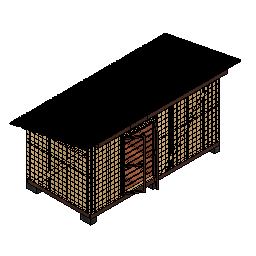
Сарай v19 (Autodesk Fusion 360 design; units mm, degrees)
Autodesk Fusion 360 part; units mm, degrees
note: some values were not read from the file. Chosen so that the rebuilt part matches the saved one: which bodies a step acts on; which face or edge a step refers to; where a step ends.
(part 1 of 2)
sketch "Sketch1" plane through (0, 0, 0) normal (0, 0, 1) x (1, 0, 0) in component "Обвязка"
  line L0 (0, 0) -> (5, 0)
  line L1 (5, 0) -> (5, 15)
  line L2 (5, 15) -> (0, 15)
  line L3 (0, 15) -> (0, 0)
  line L4 (0, 15) -> (-240, 15)
  line L5 (-240, 15) -> (-240, 0)
  line L6 (-240, 0) -> (0, 0)
  line L7 (0, 0) -> (0, 15)
  line L8 (-240, 15) -> (-245, 15)
  line L9 (-245, 15) -> (-245, 0)
  line L10 (-245, 0) -> (-240, 0)
  line L11 (-240, 0) -> (-240, 15)
  line L12 (-240, 15) -> (-235, 15)
  line L13 (-235, 15) -> (-235, 0)
  line L14 (-235, 0) -> (-240, 0)
  line L15 (-240, 0) -> (-240, 15)
  line L16 (0, 15) -> (-5, 15)
  line L17 (-5, 15) -> (-5, 0)
  line L18 (-5, 0) -> (0, 0)
  line L19 (0, 0) -> (0, 15)
  dimension "d1" = 5
  dimension "d2" = 15
  dimension "d3" = 240
  dimension "d4" = 15
  dimension "d5" = 5
  dimension "d6" = 15
  dimension "d7" = 5
  dimension "d8" = 15
  dimension "d9" = 5
  dimension "d10" = 15
  constraint horizontal L0
  constraint vertical L1
  constraint horizontal L2
  constraint vertical L3
  constraint coincident L0.start L3.end
  constraint horizontal L4
  constraint vertical L5
  constraint horizontal L6
  constraint vertical L7
  constraint horizontal L8
  constraint vertical L9
  constraint horizontal L10
  constraint vertical L11
  constraint horizontal L12
  constraint vertical L13
  constraint horizontal L14
  constraint vertical L15
  constraint horizontal L16
  constraint vertical L17
  constraint horizontal L18
  constraint vertical L19
  measures "d1" distance of L0.start L0.end
  measures "d2" distance of L0.start L2.end
  measures "d3" distance of L2.end L4.end
  measures "d4" distance of L2.end L0.start
  measures "d5" distance of L4.end L8.end
  measures "d6" distance of L4.end L5.end
  measures "d7" distance of L4.end L12.end
  measures "d8" distance of L4.end L5.end
  measures "d9" distance of L2.end L16.end
  measures "d10" distance of L2.end L0.start
extrude "Extrude1" add sketch "Sketch1" against normal blind 500 contours L0 L1 L2 L3 L7 L19 makes body 1 in component "Обвязка"
extrude "Extrude2" add sketch "Sketch1" against normal blind 500 separate body contours L5 L8 L9 L10 L11 L15 makes body 2 in component "Обвязка"
extrude "Extrude3" add sketch "Sketch1" against normal blind 5 separate body contours L3 L4 L6 L7 L16 L17 L18 L19 | L4 L6 L13 L17 | L4 L5 L6 L11 L12 L13 L14 L15 makes body 3 in component "Обвязка"
copy_body "CopyPasteBodies1" bodies 3 makes body 4 in component "Обвязка"
move_body "Move1" bodies 4 to x (1, 0, 0) y (0, 1, 0) z (0, 0, 1) at (0, 0, -495) in component "Обвязка"
extrude "Extrude4" add sketch "Sketch1" against normal blind 490 from surface at -5 separate body contours L3 L4 L6 L7 L16 L17 L18 L19 makes body 5 in component "Обвязка"
copy_body "CopyPasteBodies2" bodies 5 makes body 6 in component "Обвязка"
move_body "Move2" bodies 6 to x (1, 0, 0) y (0, 1, 0) z (0, 0, 1) at (-235, 0, 0) in component "Обвязка"
extrude "Extrude5" add sketch "Sketch1" against normal blind 5 from surface at -5 separate body contours L4 L6 L13 L17 makes body 7 in component "Обвязка"
copy_body "CopyPasteBodies3" bodies 7 makes body 8 in component "Обвязка"
move_body "Move3" bodies 8 to x (1, 0, 0) y (0, 1, 0) z (0, 0, 1) at (0, 0, -485) in component "Обвязка"
sketch "Sketch3" plane through (-235, 0, 0) normal (1, 0, 0) x (0, 0, -1) in component "Обвязка"
  line L0 (5, 15) -> (5, 0)
  line L1 (5, 0) -> (495, 0)
  line L2 (495, 0) -> (495, 15)
  line L3 (495, 15) -> (5, 15)
  point P0 (250, 15)
  constraint midpoint L3 P0
copy_body "CopyPasteBodies4" bodies 7 makes body 9 in component "Обвязка"
move_body "Move4" bodies 9 to x (1, 0, 0) y (0, 1, 0) z (0, 0, 1) at (0, 0, -240) in component "Обвязка"
copy_body "CopyPasteBodies5" bodies 9 makes body 10 in component "Обвязка"
move_body "Move5" bodies 10 to x (1, 0, 0) y (0, 1, 0) z (0, 0, 1) at (0, 0, -5) in component "Обвязка"
sketch "Sketch1 (2)" plane through (0, 0, 0) normal (0, 1, 0) x (1, 0, 0) in component "Фундамент"
  line L0 (-245, 0) -> (-205, 0)
  line L1 (-205, 0) -> (-205, 20)
  line L2 (-205, 20) -> (-245, 20)
  line L3 (-245, 20) -> (-245, 0)
  point P0 (-245, 0)
  dimension "d23" = 40
  dimension "d24" = 20
  constraint horizontal L0
  constraint vertical L1
  constraint horizontal L2
  constraint vertical L3
  constraint coincident P0 L0.start
  measures "d23" distance of P0 L0.end
  measures "d24" distance of P0 L2.end
extrude "Extrude1'" add sketch "Sketch1 (2)" against normal blind 20 separate body makes body 11 in component "Фундамент"
copy_body "CopyPasteBodies1'" bodies 11 makes body 12 in component "Фундамент"
move_body "Move1'" bodies 12 to x (1, 0, 0) y (0, 1, 0) z (0, 0, 1) at (210, 0, 0) in component "Фундамент"
copy_body "CopyPasteBodies2'" bodies 12 makes body 13 in component "Фундамент"
move_body "Move2'" bodies 13 to x (1, 0, 0) y (0, 1, 0) z (0, 0, 1) at (0, 0, -480) in component "Фундамент"
copy_body "CopyPasteBodies3'" bodies 11 makes body 14 in component "Фундамент"
move_body "Move3'" bodies 14 to x (1, 0, 0) y (0, 1, 0) z (0, 0, 1) at (0, 0, -480) in component "Фундамент"
copy_body "CopyPasteBodies4'" bodies 13 makes body 15 in component "Фундамент"
move_body "Move4'" bodies 15 to x (1, 0, 0) y (0, 1, 0) z (0, 0, 1) at (0, 0, 240) in component "Фундамент"
copy_body "CopyPasteBodies5'" bodies 15 makes body 16 in component "Фундамент"
move_body "Move5'" bodies 16 to x (1, 0, 0) y (0, 1, 0) z (0, 0, 1) at (-210, 0, 0) in component "Фундамент"
sketch "Sketch1 (3)" plane through (0, 0, 0) normal (0, 0, 1) x (1, 0, 0)
  line L0 (5, 15) -> (5, 295) construction
  line L1 (-245, 15) -> (-245, 295) construction
  line L2 (-302.9339, 205.9567) -> (-298.7516, 205.9567) construction
  line L3 (-298.7516, 205.9567) -> (44.8179, 272.7398) construction
  line L4 (-297.3309, 190.9521) -> (46.2386, 257.7352) construction
  point P0 (5, 15)
  point P1 (-245, 15)
  point P2 (5, 265)
  point P3 (5, 265)
  point P4 (5, 249.7192)
  point P5 (-245, 201.1242)
  point P6 (-245, 216.4049)
  dimension "d29" = 280
  dimension "d30" = 280
  dimension "d31" = 350
  dimension "d32" = 79
  dimension "d33" = 250
  dimension "d34" = 15
  constraint coincident P0 L0.start
  constraint vertical L0
  constraint coincident P1 L1.start
  constraint parallel L0 L1
  constraint perpendicular L1 L2
  constraint coincident L0 P3
  constraint coincident L3 P3
  constraint equal L3 L4
  constraint parallel L3 L4
  constraint coincident L4 P4
  constraint coincident L0 P4
  constraint coincident L4 P5
  constraint coincident L1 P5
  constraint coincident L1 P6
  constraint coincident L3 P6
  measures "d29" distance of P0 L0.end
  measures "d30" distance of P1 L1.end
  measures "d31" distance of L2.end L3.end
  measures "d32" angle of L0 L3
  measures "d33" distance of P0 P2
  measures "d34" distance of L3 L4
sketch "Sketch6" plane through (0, 0, 0) normal (0, 0, 1) x (1, 0, 0) in component "ЛицеваяСтена"
  line L0 (5, 15) -> (-5, 15)
  line L1 (-5, 15) -> (-5, 20)
  line L2 (-5, 20) -> (5, 20)
  line L3 (5, 20) -> (5, 15)
  line L4 (5, 15) -> (5, 264.9355) construction
  line L5 (5, 250.7192) -> (-5, 250.7192)
  line L6 (-5, 250.7192) -> (-5, 245.7192)
  line L7 (-5, 245.7192) -> (5, 245.7192)
  line L8 (5, 245.7192) -> (5, 250.7192)
  line L9 (5, 245.7192) -> (-5, 245.7192)
  line L10 (-5, 245.7192) -> (-5, 20)
  line L11 (-5, 20) -> (5, 20)
  line L12 (5, 20) -> (5, 245.7192)
  point P0 (5, 15)
  point P1 (5, 249.7192)
  point P2 (5, 250.7192)
  dimension "d42" = 10
  dimension "d43" = 5
  dimension "d44" = 1
  dimension "d45" = 10
  dimension "d46" = 5
  constraint horizontal L0
  constraint vertical L1
  constraint horizontal L2
  constraint vertical L3
  constraint coincident P0 L0.start
  constraint perpendicular L0 L4
  constraint coincident L4 P2
  constraint horizontal L5
  constraint vertical L6
  constraint horizontal L7
  constraint vertical L8
  constraint coincident P2 L5.start
  constraint horizontal L9
  constraint vertical L10
  constraint horizontal L11
  constraint vertical L12
  measures "d42" distance of P0 L0.end
  measures "d43" distance of P0 L2.end
  measures "d44" distance of P1 L5.start
  measures "d45" distance of P2 L5.end
  measures "d46" distance of P2 L7.end
extrude "Extrude2'" add sketch "Sketch6" against normal blind 500 separate body contours L0 L1 L2 L3 L11 makes body 17 in component "ЛицеваяСтена"
extrude "Extrude3'" add sketch "Sketch6" against normal blind 500 separate body contours L5 L6 L7 L8 L9 makes body 18 in component "ЛицеваяСтена"
extrude "Extrude4'" add sketch "Sketch6" against normal blind 5 separate body contours L2 L7 L9 L10 L11 L12 makes body 19 in component "ЛицеваяСтена"
pattern_linear "R-Pattern1" count 9 spacing 61.875 along (0, 0, -1) of bodies 19 makes body 20 at (-1.6667, 95.2397, -61.875) makes body 21 at (-1.6667, 95.2397, -123.75) makes body 22 at (-1.6667, 95.2397, -185.625) makes body 23 at (-1.6667, 95.2397, -247.5) makes body 24 at (-1.6667, 95.2397, -309.375) makes body 25 at (-1.6667, 95.2397, -371.25) makes body 26 at (-1.6667, 95.2397, -433.125) makes body 27 at (-1.6667, 95.2397, -495) in component "ЛицеваяСтена"
box "BoxPrimitive2" add length 250 width 125 height 1 placed x (0, 1, 0) y (0, 0, -1) z (-1, 0, 0) at (-5, 15, 0) separate body makes body 28 in component "ЛицеваяСтена"
sketch "Sketch9" plane through (5, 0, 0) normal (1, 0, 0) x (0, 0, -1) in component "ЛицеваяСтена"
  line L0 (0, 20) -> (0, 15)
  line L1 (0, 15) -> (500, 15)
  line L2 (500, 15) -> (500, 20)
  line L3 (500, 20) -> (0, 20)
  line L4 (120, 20) -> (120, 235) construction
  line L5 (255, 20) -> (255, 235) construction
  line L6 (120, 210) -> (255, 210) construction
  line L7 (120, 220) -> (255, 220) construction
  line L8 (185, 210) -> (185, 220) construction
  line L9 (0, 245.7192) -> (500, 245.7192)
  line L10 (492.3524, 260.7433) -> (289.7663, 14.3411) construction
  line L11 (467.0712, 253.613) -> (259.1771, 0.7549) construction
  line L12 (0, 250.7192) -> (500, 250.7192) construction
  line L13 (0, 20) -> (500, 20) construction
  line L14 (0, 15) -> (500, 15) construction
  line L15 (270.8891, 15) -> (290.308, 15)
  line L16 (290.308, 15) -> (484.1109, 250.7192)
  line L17 (484.1109, 250.7192) -> (464.692, 250.7192)
  line L18 (464.692, 250.7192) -> (270.8891, 15)
  point P0 (125, 20)
  point P1 (250, 20)
  point P2 (0, 20)
  point P3 (125, 20)
  point P4 (120, 20)
  point P5 (255, 20)
  point P6 (120, 210)
  point P7 (187.5, 210)
  point P8 (185, 210)
  point P9 (120, 220)
  point P10 (185, 220)
  point P11 (275, 20)
  point P12 (480, 245.7192)
  point P13 (495, 245.7192)
  point P14 (480, 245.7192)
  point P15 (275, 20)
  dimension "d67" = 125
  dimension "d68" = 125
  dimension "d69" = 5
  dimension "d70" = 5
  dimension "d71" = 215
  dimension "d72" = 215
  dimension "d73" = 190
  dimension "d79" = 2.5
  dimension "d80" = 10
  dimension "d96" = 20
  dimension "d97" = 15
  dimension "d98" = 15
  constraint coincident L3 P3
  constraint coincident L3 P1
  constraint coincident P2 L0.start
  constraint coincident P3 P0
  constraint coincident L3 P4
  constraint coincident L3 P5
  constraint coincident P4 L4.start
  constraint perpendicular L3 L4
  constraint coincident P5 L5.start
  constraint perpendicular L3 L5
  constraint coincident L4 P6
  constraint coincident P6 L6.start
  constraint coincident L5 L6.end
  constraint perpendicular L5 L6
  constraint midpoint L6 P7
  constraint coincident L6 P8
  constraint coincident L4 P9
  constraint coincident P9 L7.start
  constraint coincident L5 L7.end
  constraint perpendicular L5 L7
  constraint coincident P8 L8.start
  constraint coincident L7 P10
  constraint perpendicular L7 L8
  constraint coincident P10 L8.end
  constraint coincident L3 P15
  constraint coincident L9 P14
  constraint parallel L10 L11
  constraint coincident L10 P14
  constraint coincident L11 P15
  constraint coincident P14 P12
  constraint coincident P15 P11
  constraint coincident L11 L15.start
  constraint coincident L14 L15.start
  constraint coincident L10 L15.end
  constraint coincident L14 L15.end
  constraint coincident L10 L16.end
  constraint coincident L12 L16.end
  constraint coincident L11 L17.end
  constraint coincident L12 L17.end
  measures "d67" distance of P2 P3
  measures "d68" distance of P3 P1
  measures "d69" distance of P3 P4
  measures "d70" distance of P1 P5
  measures "d71" distance of P4 L4.end
  measures "d72" distance of P5 L5.end
  measures "d73" distance of P4 P6
  measures "d79" distance of P7 P8
  measures "d80" distance of P6 P9
  measures "d96" distance of P5 P15
  measures "d97" distance of P14 P13
  measures "d98" distance of L10 L11
move_body "Move2''" bodies 21 to x (1, 0, 0) y (0, 1, 0) z (0, 0, 1) at (0, 0, 3.75) in component "ЛицеваяСтена"
move_body "Move3''" bodies 23 to x (1, 0, 0) y (0, 1, 0) z (0, 0, 1) at (0, 0, -2.5) in component "ЛицеваяСтена"
move_body "Move4''" bodies 22 to x (1, 0, 0) y (0, 1, 0) z (0, 0, 1) at (0, 0, 70.625) in component "ЛицеваяСтена"
copy_body "CopyPasteBodies2''" bodies 22 makes body 29 in component "ЛицеваяСтена"
move_body "Move5''" bodies 29 to x (1, 0, 0) y (0, 1, 0) z (0, 0, 1) at (0, 0, -140) in component "ЛицеваяСтена"
box "BoxPrimitive4" add length 5 width 10 height 135 placed x (0, 1, 0) y (1, 0, 0) z (0, 0, -1) at (-5, 210.0714, -120) separate body makes body 30 in component "ЛицеваяСтена"
copy_body "CopyPasteBodies3''" bodies 30 makes body 31 in component "ЛицеваяСтена"
move_body "Move6" bodies 31 to x (1, 0, 0) y (0, 1, 0) z (0, 0, 1) at (0, 5, 0) in component "ЛицеваяСтена"
combine "Combine1" operation cut target body 21 tool bodies 30 31 keep tools makes body 32 at (-1.6667, 237.17, -120) in component "ЛицеваяСтена"
combine "Combine2" operation cut target body 23 tool bodies 30 31 keep tools makes body 33 at (-1.6667, 146.7143, -250) in component "ЛицеваяСтена"
copy_body "CopyPasteBodies4''" bodies 32 makes body 34 in component "ЛицеваяСтена"
move_body "Move7" bodies 34 to x (1, 0, 0) y (0, 1, 0) z (0, 0, 1) at (0, 0, -65) in component "ЛицеваяСтена"
sketch "Sketch1 (4)" plane through (0, 0, 0) normal (0, 0, 1) x (1, 0, 0) in component "ЗадняяСтена"
  line L0 (-245, 15) -> (-245, 230.3796) construction
  line L1 (-297.3309, 190.9521) -> (46.2386, 257.7352) construction
  line L2 (-245, 15) -> (-235, 15)
  line L3 (-235, 15) -> (-235, 20)
  line L4 (-235, 20) -> (-245, 20)
  line L5 (-245, 20) -> (-245, 15)
  line L6 (-235, 20) -> (-235, 230.5911) construction
  line L7 (-235, 204.068) -> (-245, 204.068)
  line L8 (-245, 204.068) -> (-245, 199.068)
  line L9 (-245, 199.068) -> (-235, 199.068)
  line L10 (-235, 199.068) -> (-235, 204.068)
  line L11 (-245, 199.068) -> (-235, 199.068)
  line L12 (-235, 199.068) -> (-235, 20)
  line L13 (-235, 20) -> (-245, 20)
  line L14 (-245, 20) -> (-245, 199.068)
  point P0 (-245, 15)
  point P1 (-245, 201.1242)
  point P2 (-235, 203.068)
  point P3 (-235, 204.068)
  dimension "d81" = 10
  dimension "d82" = 5
  dimension "d83" = 1
  dimension "d84" = 10
  dimension "d85" = 5
  constraint coincident P0 L0.start
  constraint vertical L0
  constraint horizontal L2
  constraint vertical L3
  constraint horizontal L4
  constraint vertical L5
  constraint perpendicular L4 L6
  constraint coincident L1 P2
  constraint coincident L6 P2
  constraint coincident L6 P3
  constraint horizontal L7
  constraint vertical L8
  constraint horizontal L9
  constraint vertical L10
  constraint coincident P3 L7.start
  constraint horizontal L11
  constraint vertical L12
  constraint horizontal L13
  constraint vertical L14
  measures "d81" distance of P0 L2.end
  measures "d82" distance of P0 L4.end
  measures "d83" distance of P2 P3
  measures "d84" distance of P3 L7.end
  measures "d85" distance of P3 L9.end
extrude "Extrude1''" add sketch "Sketch1 (4)" against normal blind 500 separate body contours L2 L3 L4 L5 L13 makes body 35 in component "ЗадняяСтена"
extrude "Extrude2''" add sketch "Sketch1 (4)" against normal blind 500 separate body contours L7 L8 L9 L10 L11 makes body 36 in component "ЗадняяСтена"
extrude "Extrude3''" add sketch "Sketch1 (4)" against normal blind 5 separate body contours L4 L9 L11 L12 L13 L14 makes body 37 in component "ЗадняяСтена"
sketch "Sketch2" plane through (-245, 0, 0) normal (-1, 0, 0) x (0, 0, 1) in component "ЗадняяСтена"
  line L0 (0, 15) -> (0, 20)
  line L1 (0, 20) -> (-500, 20)
  line L2 (-500, 20) -> (-500, 15)
  line L3 (-500, 15) -> (0, 15)
  line L4 (-185, 220.0714) -> (-185, 176.1812) construction
  line L5 (0, 199.068) -> (-500, 199.068) construction
  line L6 (0, 20) -> (-500, 20)
  line L7 (0, 199.068) -> (-500, 199.068)
  line L8 (0, 204.068) -> (-500, 204.068)
  line L9 (-466.0975, 206.5456) -> (-261.8081, 12.2071) construction
  line L10 (-487.598, 206.2959) -> (-282.9377, 11.6045) construction
  line L11 (-230.99, 2.9641) -> (-230.99, 3.2571) construction
  line L12 (-230.99, 3.2571) -> (-11.0284, 207.3942) construction
  line L13 (-22.6395, 217.0828) -> (-243.8333, 11.8022) construction
  line L14 (-485.256, 204.068) -> (-463.4929, 204.068)
  line L15 (-463.4929, 204.068) -> (-264.744, 15)
  line L16 (-264.744, 15) -> (-286.5071, 15)
  line L17 (-286.5071, 15) -> (-485.256, 204.068)
  line L18 (-240.3876, 15) -> (-218.3368, 15)
  line L19 (-218.3368, 15) -> (-14.6124, 204.068)
  line L20 (-14.6124, 204.068) -> (-36.6632, 204.068)
  line L21 (-36.6632, 204.068) -> (-240.3876, 15)
  point P0 (-125, 20)
  point P1 (-250, 20)
  point P2 (-185, 220.0714)
  point P3 (-185, 199.068)
  point P4 (-270, 20)
  point P5 (-235, 20)
  point P6 (-480, 199.068)
  point P7 (-20, 199.068)
  point P8 (-5, 199.068)
  point P9 (-480, 199.068)
  point P10 (-270, 20)
  point P11 (-20, 199.068)
  point P12 (-235, 20)
  point P13 (-247.5, 20)
  dimension "d103" = 20
  dimension "d104" = 15
  dimension "d105" = 20
  dimension "d106" = 15
  dimension "d107" = 15
  dimension "d108" = 15
  dimension "d173" = 252.5
  constraint coincident P2 L4.start
  constraint vertical L4
  constraint coincident L4 P3
  constraint coincident L5 P3
  constraint coincident L1 P10
  constraint coincident L1 P12
  constraint coincident L5 P9
  constraint coincident L5 P11
  constraint parallel L9 L10
  constraint coincident L10 P9
  constraint coincident L9 P10
  constraint coincident P9 P6
  constraint coincident P10 P4
  constraint perpendicular L3 L11
  constraint parallel L12 L13
  constraint coincident L12 P11
  constraint coincident L13 P12
  constraint coincident P11 P7
  constraint coincident P12 P5
  constraint coincident L10 L14.start
  constraint coincident L8 L14.start
  constraint coincident L9 L14.end
  constraint coincident L8 L14.end
  constraint coincident L9 L15.end
  constraint coincident L3 L15.end
  constraint coincident L3 L16.end
  constraint coincident L10 L16.end
  constraint coincident L3 L18.start
  constraint coincident L13 L18.start
  constraint coincident L12 L18.end
  constraint coincident L3 L18.end
  constraint coincident L8 L19.end
  constraint coincident L12 L19.end
  constraint coincident L13 L20.end
  constraint coincident L8 L20.end
  constraint coincident L1 P13
  measures "d103" distance of P1 P10
  measures "d104" distance of P1 P12
  measures "d105" distance of L5.end P9
  measures "d106" distance of P11 P8
  measures "d107" distance of L9 L10
  measures "d108" distance of L12 L13
  measures "d173" distance of L1.end P13
pattern_linear "R-Pattern1'" count 9 spacing 61.875 along (0, 0, -1) of bodies 37 makes body 38 at (-241.6667, 139.3787, -61.875) makes body 39 at (-241.6667, 139.3787, -123.75) makes body 40 at (-241.6667, 139.3787, -185.625) makes body 41 at (-241.6667, 139.3787, -247.5) makes body 42 at (-241.6667, 139.3787, -309.375) makes body 43 at (-241.6667, 139.3787, -371.25) makes body 44 at (-241.6667, 139.3787, -433.125) makes body 45 at (-241.6667, 139.3787, -495) in component "ЗадняяСтена"
move_body "Move1''" bodies 41 to x (1, 0, 0) y (0, 1, 0) z (0, 0, 1) at (0, 0, -2.5) in component "ЗадняяСтена"
move_body "Move2'''" bodies 39 to x (1, 0, 0) y (0, 1, 0) z (0, 0, 1) at (0, 0, 3.75) in component "ЗадняяСтена"
move_body "Move3'''" bodies 40 to x (1, 0, 0) y (0, 1, 0) z (0, 0, 1) at (0, 0, 0.625) in component "ЗадняяСтена"
extrude "Extrude5'" cut sketch "Sketch9" against normal blind 2.5 contours L3 L9 L16 L18 | L1 L3 L15 L16 L18 | L9 L16 L17 L18 bodies 17 18 24 25 26 in component "ЛицеваяСтена"
extrude "Extrude6" add sketch "Sketch9" against normal blind 2.5 separate body contours L3 L9 L16 L18 | L1 L3 L15 L16 L18 | L9 L16 L17 L18 makes body 46 in component "ЛицеваяСтена"
extrude "Extrude4''" cut sketch "Sketch2" against normal blind 2.5 contours L1 L3 L6 L18 L19 L21 | L1 L6 L7 L19 L21 | L7 L8 L19 L20 L21 | L1 L3 L6 L15 L16 L17 | L1 L6 L7 L15 L17 | L7 L8 L14 L15 L17 bodies 35 36 38 39 40 42 43 44 in component "ЗадняяСтена"
extrude "Extrude5''" add sketch "Sketch2" against normal blind 2.5 separate body contours L1 L3 L6 L15 L16 L17 | L1 L6 L7 L15 L17 | L7 L8 L14 L15 L17 makes body 47 in component "ЗадняяСтена"
extrude "Extrude6'" add sketch "Sketch2" against normal blind 2.5 separate body contours L1 L3 L6 L18 L19 L21 | L1 L6 L7 L19 L21 | L7 L8 L19 L20 L21 makes body 48 in component "ЗадняяСтена"
box "BoxPrimitive1" add length 5 width 10 height 230 placed x (0, 1, 0) y (0, 0, 1) z (1, 0, 0) at (-235, 15, -10) separate body makes body 49 in component "БоковаяСтена"
box "BoxPrimitive2'" add length 5 width 10 height 230 placed x (0, -1, 0) y (0, 0, -1) z (1, 0, 0) at (-235, 204.068, 0) separate body makes body 50 in component "БоковаяСтена"
sketch "Sketch3 (2)" plane through (0, 20, 0) normal (0, 1, 0) x (-1, 0, 0) in component "БоковаяСтена"
  line L0 (5, -10) -> (235, -10)
  line L1 (235, -10) -> (235, 0)
  line L2 (235, 0) -> (5, 0)
  line L3 (5, 0) -> (5, -10)
  line L4 (235, 0) -> (230, 0)
  line L5 (230, 0) -> (230, -10)
  line L6 (230, -10) -> (235, -10)
  line L7 (235, -10) -> (235, 0)
  dimension "d125" = 5
  dimension "d126" = 10
  constraint horizontal L4
  constraint vertical L5
  constraint horizontal L6
  constraint vertical L7
  constraint coincident L1.end L2.start
  measures "d125" distance of L1.end L4.end
  measures "d126" distance of L1.end L0.end
extrude "Extrude1'''" add sketch "Sketch3 (2)" along normal up to near side of body 50 separate body contours L0 L1 L2 L4 L5 L6 L7 makes body 51 in component "БоковаяСтена"
pattern_linear "R-Pattern1''" count 4 spacing 75 along (1, 0, 0) of bodies 51 makes body 52 at (-155, 79.6893, -3.3333) makes body 53 at (-80, 79.6893, -3.3333) makes body 54 at (-5, 79.6893, -3.3333) in component "БоковаяСтена"
sketch "Sketch4" plane through (0, 0, 0) normal (0, 0, 1) x (1, 0, 0) in component "БоковаяСтена"
  line L0 (-5, 20) -> (-235, 20)
  line L1 (-235, 20) -> (-235, 15)
  line L2 (-235, 15) -> (-5, 15)
  line L3 (-5, 15) -> (-5, 20)
  line L4 (-5, 204.068) -> (-235, 204.068)
  line L5 (-5, 199.068) -> (-235, 199.068)
  line L6 (-5, 20) -> (-235, 20)
  line L7 (-5, 15) -> (-235, 15)
  line L8 (-10.438, 214.4653) -> (-221.9216, -9.1487) construction
  line L9 (-27.6563, 218.0893) -> (-239.14, -5.5246) construction
  line L10 (-40.9171, 204.068) -> (-20.2712, 204.068)
  line L11 (-20.2712, 204.068) -> (-199.0829, 15)
  line L12 (-199.0829, 15) -> (-219.7288, 15)
  line L13 (-219.7288, 15) -> (-40.9171, 204.068)
  point P0 (-215, 20)
  point P1 (-25, 199.068)
  point P2 (-10, 199.068)
  point P3 (-230, 20)
  point P4 (-25, 199.068)
  point P5 (-215, 20)
  dimension "d133" = 15
  dimension "d134" = 15
  dimension "d135" = 15
  constraint coincident L0 P0
  constraint coincident L5 P4
  constraint parallel L8 L9
  constraint coincident L8 P4
  constraint coincident L9 P5
  constraint coincident P4 P1
  constraint coincident P0 P5
  constraint coincident L9 L10.start
  constraint coincident L4 L10.start
  constraint coincident L8 L10.end
  constraint coincident L4 L10.end
  constraint coincident L7 L11.end
  constraint coincident L8 L11.end
  constraint coincident L9 L12.end
  constraint coincident L7 L12.end
  measures "d133" distance of P4 P2
  measures "d134" distance of P0 P3
  measures "d135" distance of L8 L9
extrude "Extrude2'''" cut sketch "Sketch4" against normal blind 2.5 contours L0 L2 L6 L7 L11 L12 L13 | L0 L5 L6 L11 L13 | L4 L5 L10 L11 L13 bodies 49 50 52 53 in component "БоковаяСтена"
extrude "Extrude3'''" add sketch "Sketch4" against normal blind 2.5 separate body contours L0 L2 L6 L7 L11 L12 L13 | L0 L5 L6 L11 L13 | L4 L5 L10 L11 L13 makes body 55 in component "БоковаяСтена"
mirror "MirrorComponent1" about plane through (0, 0, 0) normal (0, 0, 1) of bodies 49 50 51 52 53 54 55 makes body 56 at (-68.118, 20, 4.1667) makes body 57 at (-170.3057, 204.068, 4.1667) makes body 58 at (-230, 79.6893, 3.3333) makes body 59 at (-155, 160.5258, 4.1667) makes body 60 at (-80, 60.3044, 4.1667) makes body 61 at (-5, 79.6893, 3.3333) makes body 62 at (-151.6667, 79.6893, 0) in component "БоковаяСтена(Mirror)"
sketch "Sketch1 (5)" plane through (-235, 0, 0) normal (1, 0, 0) x (0, 0, -1) in component "Лаги"
  line L0 (5, 15) -> (5, 0)
  line L1 (5, 0) -> (495, 0)
  line L2 (495, 0) -> (495, 15)
  line L3 (495, 15) -> (5, 15)
  line L4 (61.875, 20) -> (61.875, 0) construction
  line L5 (120, 20) -> (120, 0) construction
  line L6 (185, 20) -> (185, 0) construction
  line L7 (309.375, 20) -> (309.375, 0) construction
  line L8 (371.25, 20) -> (371.25, 0) construction
  line L9 (433.125, 20) -> (433.125, 0) construction
  line L10 (61.875, 15) -> (66.875, 15)
  line L11 (66.875, 15) -> (66.875, 5)
  line L12 (66.875, 5) -> (61.875, 5)
  line L13 (61.875, 5) -> (61.875, 15)
  point P0 (61.875, 20)
  point P1 (120, 20)
  point P2 (185, 20)
  point P3 (309.375, 20)
  point P4 (371.25, 20)
  point P5 (433.125, 20)
  point P6 (120, 15)
  point P7 (185, 15)
  point P8 (309.375, 15)
  point P9 (371.25, 15)
  point P10 (433.125, 15)
  point P11 (20, 15)
  point P12 (0, 15)
  point P13 (500, 15)
  point P14 (480, 15)
  dimension "d140" = 5
  dimension "d141" = 10
  dimension "d144" = 20
  dimension "d145" = 20
  constraint coincident P0 L4.start
  constraint coincident L1 L4.end
  constraint perpendicular L1 L4
  constraint coincident P1 L5.start
  constraint coincident L1 L5.end
  constraint perpendicular L1 L5
  constraint coincident P2 L6.start
  constraint coincident L1 L6.end
  constraint perpendicular L1 L6
  constraint coincident P3 L7.start
  constraint coincident L1 L7.end
  constraint perpendicular L1 L7
  constraint coincident P4 L8.start
  constraint coincident L1 L8.end
  constraint perpendicular L1 L8
  constraint coincident P5 L9.start
  constraint coincident L1 L9.end
  constraint perpendicular L1 L9
  constraint horizontal L10
  constraint vertical L11
  constraint horizontal L12
  constraint vertical L13
  constraint coincident L3 L10.start
  constraint coincident L4 L10.start
  constraint coincident L5 P6
  constraint coincident L3 P6
  constraint coincident L6 P7
  constraint coincident L3 P7
  constraint coincident L7 P8
  constraint coincident L3 P8
  constraint coincident L8 P9
  constraint coincident L3 P9
  constraint coincident L9 P10
  constraint coincident L3 P10
  constraint coincident L3 P11
  constraint coincident L3 P14
  measures "d140" distance of L10.start L10.end
  measures "d141" distance of L10.start L12.end
  measures "d144" distance of P11 P12
  measures "d145" distance of P13 P14
extrude "Extrude1''''" add sketch "Sketch1 (5)" along normal blind 230 separate body contours L3 L10 L11 L12 L13 makes body 63 in component "Лаги"
copy_body "CopyPasteBodies1''" bodies 63 makes body 64 in component "Лаги"
move_body "Move1'''" bodies 64 to x (1, 0, 0) y (0, 1, 0) z (0, 0, 1) at (0, 0, -58.125) in component "Лаги"
copy_body "CopyPasteBodies2'''" bodies 64 makes body 65 in component "Лаги"
move_body "Move2''''" bodies 65 to x (1, 0, 0) y (0, 1, 0) z (0, 0, 1) at (0, 0, -65) in component "Лаги"
copy_body "CopyPasteBodies3'''" bodies 65 makes body 66 in component "Лаги"
move_body "Move3''''" bodies 66 to x (1, 0, 0) y (0, 1, 0) z (0, 0, 1) at (0, 0, -124.375) in component "Лаги"
copy_body "CopyPasteBodies4'''" bodies 66 makes body 67 in component "Лаги"
move_body "Move4'''" bodies 67 to x (1, 0, 0) y (0, 1, 0) z (0, 0, 1) at (0, 0, -61.875) in component "Лаги"
copy_body "CopyPasteBodies5''" bodies 67 makes body 68 in component "Лаги"
move_body "Move5'''" bodies 68 to x (1, 0, 0) y (0, 1, 0) z (0, 0, 1) at (0, 0, -61.875) in component "Лаги"
copy_body "CopyPasteBodies6" bodies 63 makes body 69 in component "Лаги"
move_body "Move6'" bodies 69 to x (1, 0, 0) y (0, 1, 0) z (0, 0, 1) at (0, 0, 41.875) in component "Лаги"
copy_body "CopyPasteBodies7" bodies 68 makes body 70 in component "Лаги"
move_body "Move7'" bodies 70 to x (1, 0, 0) y (0, 1, 0) z (0, 0, 1) at (0, 0, -41.875) in component "Лаги"
sketch "Sketch1 (6)" plane through (0, 0, 0) normal (0, 0, 1) x (1, 0, 0) in component "Стропила"
  line L0 (-298.7516, 205.9567) -> (44.8179, 272.7398)
  line L1 (-297.3309, 190.9521) -> (46.2386, 257.7352)
  line L2 (-259.4542, 261.2143) -> (-259.4542, 7.593) construction
  line L3 (35, 295.2761) -> (35, -0.5469) construction
  line L4 (5, 15) -> (5, 295) construction
  line L5 (-259.4882, 213.5887) -> (-256.626, 198.8643)
  line L6 (-259.4882, 213.5887) -> (35, 270.8314)
  line L7 (35, 270.8314) -> (35, 255.5507)
  line L8 (35, 255.5507) -> (-256.626, 198.8643)
  line L9 (-245, 199.068) -> (-235, 199.068)
  line L10 (-235, 199.068) -> (-235, 204.068)
  line L11 (-235, 204.068) -> (-245, 204.068)
  line L12 (-245, 204.068) -> (-245, 199.068)
  line L13 (-245, 201.1242) -> (-245, 204.068)
  line L14 (-235, 204.068) -> (-234.9283, 203.0819)
  line L15 (-45.6459, 199.068) -> (-40.9171, 204.068)
  line L16 (-40.9171, 204.068) -> (-235, 204.068)
  line L17 (-235, 204.068) -> (-235, 199.068)
  line L18 (-235, 199.068) -> (-45.6459, 199.068)
  line L19 (-235, 204.068) -> (-229.8554, 204.068)
  point P0 (-259.4882, 213.5887)
  point P1 (35, 270.8314)
  dimension "d146" = 300
  dimension "d147" = 30
  constraint coincident L0 P0
  constraint coincident L0 P1
  constraint vertical L2
  constraint parallel L2 L3
  constraint coincident P1 L3
  constraint coincident P0 L5.start
  constraint coincident L1 L5.end
  constraint perpendicular L1 L5
  constraint coincident P1 L6.end
  constraint coincident L3 L7.end
  constraint coincident L1 L7.end
  constraint coincident L1 L13.start
  constraint coincident L12 L13.start
  constraint coincident L11.end L12.start
  constraint coincident L10.end L11.start
  constraint coincident L1 L14.end
  constraint coincident L8 L19.end
  constraint coincident L16 L19.end
  measures "d146" distance of P0 P1
  measures "d147" distance of L3 L4
extrude "Extrude1'''''" add sketch "Sketch1 (6)" against normal blind 5 separate body contours L0 L1 L5 L6 L7 L8 L11 L12 L13 L16 L19 | L1 L8 L14 L16 L19 makes body 71 in component "Стропила"
pattern_linear "R-Pattern1'''" count 9 spacing 61.875 along (0, 0, -1) of bodies 71 makes body 72 at (-151.4479, 229.496, -61.875) makes body 73 at (-151.4479, 229.496, -123.75) makes body 74 at (-151.4479, 229.496, -185.625) makes body 75 at (-151.4479, 229.496, -247.5) makes body 76 at (-151.4479, 229.496, -309.375) makes body 77 at (-151.4479, 229.496, -371.25) makes body 78 at (-151.4479, 229.496, -433.125) makes body 79 at (-151.4479, 229.496, -495) in component "Стропила"
sketch "Sketch2 (2)" plane through (-245, 0, 0) normal (-1, 0, 0) x (0, 0, 1) in component "Стропила"
  line L0 (-66.875, 176.0297) -> (-61.875, 180.6699)
  line L1 (-61.875, 180.6699) -> (-61.875, 199.068)
  line L2 (-61.875, 199.068) -> (-66.875, 199.068)
  line L3 (-66.875, 199.068) -> (-66.875, 176.0297)
  line L4 (-255, 199.068) -> (-255, 207.4684) construction
  line L5 (-120, 199.068) -> (-120, 207.4684) construction
  line L6 (-463.4929, 204.068) -> (-458.2369, 199.068) construction
  line L7 (-458.2369, 199.068) -> (-42.0508, 199.068) construction
  line L8 (-42.0508, 199.068) -> (-36.6632, 204.068) construction
  line L9 (-36.6632, 204.068) -> (-463.4929, 204.068) construction
  point P0 (-120, 199.068)
  point P1 (-255, 199.068)
  point P2 (-255, 204.068)
  point P3 (-120, 204.068)
  constraint coincident P1 L4.start
  constraint vertical L4
  constraint coincident P0 L5.start
  constraint parallel L4 L5
  constraint coincident L4 P2
  constraint coincident L9 P2
  constraint coincident L5 P3
  constraint coincident L9 P3
move_body "Move1''''" bodies 73 to x (1, 0, 0) y (0, 1, 0) z (0, 0, 1) at (0, 0, 3.75) in component "Стропила"
move_body "Move2'''''" bodies 75 to x (1, 0, 0) y (0, 1, 0) z (0, 0, 1) at (0, 0, -2.5) in component "Стропила"
combine "Combine1'" operation cut target body 71 tool bodies 50 keep tools in component "Стропила"
combine "Combine2'" operation cut target body 79 tool bodies 57 body 57 seen with x (1, 0, 0) y (0, 1, 0) z (0, 0, 1) at (0, 0, -500) keep tools in component "Стропила"
box "BoxPrimitive1'" add length 480 width 15 height 2.5 placed x (0, 0, -1) y (-1, 0, 0) z (0, 1, 0) at (-220, 15, -10) separate body makes body 80 in component "Пол"
pattern_linear "R-Pattern1''''" count 13 spacing 17.9167 along (1, 0, 0) of bodies 80 makes body 81 at (-212.0833, 15, -170) makes body 82 at (-194.1667, 15, -170) makes body 83 at (-176.25, 15, -170) makes body 84 at (-158.3333, 15, -170) makes body 85 at (-140.4167, 15, -170) makes body 86 at (-122.5, 15, -170) makes body 87 at (-104.5833, 15, -170) makes body 88 at (-86.6667, 15, -170) makes body 89 at (-68.75, 15, -170) makes body 90 at (-50.8333, 15, -170) makes body 91 at (-32.9167, 15, -170) makes body 92 at (-15, 15, -170) in component "Пол"
combine "Combine3" operation cut target body 71 tool bodies 18 keep tools in component "Стропила"
combine "Combine4" operation cut target body 72 tool bodies 18 keep tools in component "Стропила"
combine "Combine5" operation cut target body 73 tool bodies 18 keep tools in component "Стропила"
combine "Combine6" operation cut target body 74 tool bodies 18 keep tools in component "Стропила"
combine "Combine7" operation cut target body 75 tool bodies 18 keep tools in component "Стропила"
combine "Combine8" operation cut target body 76 tool bodies 18 keep tools in component "Стропила"
combine "Combine9" operation cut target body 77 tool bodies 18 keep tools in component "Стропила"
combine "Combine10" operation cut target body 78 tool bodies 18 keep tools in component "Стропила"
combine "Combine11" operation cut target body 79 tool bodies 18 keep tools in component "Стропила"
sketch "Sketch1 (7)" plane through (-49.4533, 254.4153, 0) normal (-0.190809, 0.981627, 0) x (0, 0, 1) in component "Обрешетка"
  line L0 (0, -213.966) -> (0, 86.034)
  line L1 (0, 86.034) -> (-5, 86.034)
  line L2 (-5, 86.034) -> (-5, -213.966)
  line L3 (-5, -213.966) -> (0, -213.966)
  line L4 (0, -213.966) -> (-500, -213.966) construction
  line L5 (-500, -213.966) -> (-500, -198.966) construction
  line L6 (-500, -198.966) -> (0, -198.966) construction
  line L7 (0, -198.966) -> (0, -213.966) construction
  line L8 (0, -198.966) -> (-500, -213.966) construction
  line L9 (-550, -198.966) -> (50, -198.966)
  line L10 (50, -198.966) -> (50, -213.966)
  line L11 (50, -213.966) -> (-550, -213.966)
  line L12 (-550, -213.966) -> (-550, -198.966)
  line L13 (-550, -198.966) -> (50, -213.966) construction
  line L14 (50, -198.966) -> (-550, -213.966) construction
  point P0 (-500, -213.966)
  point P1 (0, -213.966)
  point P2 (0, 86.034)
  point P3 (-500, 86.034)
  point P4 (-250, -206.466)
  point P5 (-250, -206.466)
  point P6 (0, -198.966)
  dimension "d163" = 500
  dimension "d164" = 15
  dimension "d165" = 600
  dimension "d166" = 15
  constraint horizontal L4
  constraint vertical L5
  constraint horizontal L6
  constraint vertical L7
  constraint coincident P1 L0.start
  constraint coincident P0 L4.end
  constraint midpoint L8 P5
  constraint horizontal L9
  constraint perpendicular L9 L10
  constraint parallel L9 L11
  constraint parallel L10 L12
  constraint coincident L13 P5
  constraint coincident L14 P5
  constraint coincident P5 P4
  constraint coincident P6 L6.end
  measures "d163" distance of P1 P0
  measures "d164" distance of P1 P6
  measures "d165" distance of L10.end L11.end
  measures "d166" distance of L9.end L10.end
extrude "Extrude1''''''" add sketch "Sketch1 (7)" along normal blind 2.5 separate body contours L0 L2 L3 L9 L11 | L0 L9 L10 L11 | L2 L9 L11 L12 makes body 93 in component "Обрешетка"
copy_body "CopyPasteBodies1'''" bodies 93 makes body 94 in component "Обрешетка"
move_body "Move1'''''" bodies 94 to x (1, 0, 0) y (0, 1, 0) z (0, 0, 1) at (14.7244, 2.8621, 0) in component "Обрешетка"
copy_body "CopyPasteBodies2''''" bodies 93 makes body 95 in component "Обрешетка"
move_body "Move2''''''" bodies 95 to x (1, 0, 0) y (0, 1, 0) z (0, 0, 1) at (279.7637, 54.3806, 0) in component "Обрешетка"
copy_body "CopyPasteBodies3''''" bodies 93 makes body 96 in component "Обрешетка"
move_body "Move3'''''" bodies 96 to x (1, 0, 0) y (0, 1, 0) z (0, 0, 1) at (265.0393, 51.5184, 0) in component "Обрешетка"
pattern_linear "R-Pattern1'''''" count 8 spacing 32.5 along (0.981627, 0.190809, 0) of bodies 94 makes body 97 at (-207.9527, 223.6062, -368.3333) makes body 98 at (-176.0498, 229.8075, -368.3333) makes body 99 at (-144.147, 236.0088, -368.3333) makes body 100 at (-112.2441, 242.2101, -368.3333) makes body 101 at (-80.3412, 248.4114, -186.6667) makes body 102 at (-48.4383, 254.6126, -368.3333) makes body 103 at (-16.5354, 260.8139, -368.3333) in component "Обрешетка"
delete_body "RemoveBody4" bodies 28 in component "ЛицеваяСтена"
move_body "Move4''''" bodies 41 to x (1, 0, 0) y (0, 1, 0) z (0, 0, 1) at (0, 0, 2.5) in component "ЗадняяСтена"
sketch "Sketch1 (8)" plane through (84.4533, 16.4161, 0) normal (0.981627, 0.190809, 0) x (0, 0, -1) in component "Крыша"
  line L0 (550, 259.1772) -> (550, 261.6772)
  line L1 (-49.25, 261.6772) -> (-47.5, 261.6772)
  line L2 (-47.5, 261.6772) -> (-45.75, 261.6772)
  line L3 (-45.75, 261.6772) -> (-44.25, 263.7772)
  line L4 (-44.25, 263.7772) -> (-40.75, 263.7772)
  line L5 (-40.75, 263.7772) -> (-39.25, 261.6772)
  line L6 (-39.25, 261.6772) -> (-37.5, 261.6772)
  line L7 (-37.5, 261.6772) -> (-35.75, 261.6772)
  line L8 (-35.75, 261.6772) -> (-34.25, 263.7772)
  line L9 (-34.25, 263.7772) -> (-30.75, 263.7772)
  line L10 (-30.75, 263.7772) -> (-29.25, 261.6772)
  line L11 (-29.25, 261.6772) -> (-27.5, 261.6772)
  line L12 (-27.5, 261.6772) -> (-25.75, 261.6772)
  line L13 (-25.75, 261.6772) -> (-24.25, 263.7772)
  line L14 (-24.25, 263.7772) -> (-20.75, 263.7772)
  line L15 (-20.75, 263.7772) -> (-19.25, 261.6772)
  line L16 (-19.25, 261.6772) -> (-17.5, 261.6772)
  line L17 (-17.5, 261.6772) -> (-15.75, 261.6772)
  line L18 (-15.75, 261.6772) -> (-14.25, 263.7772)
  line L19 (-14.25, 263.7772) -> (-10.75, 263.7772)
  line L20 (-10.75, 263.7772) -> (-9.25, 261.6772)
  line L21 (-9.25, 261.6772) -> (-7.5, 261.6772)
  line L22 (-7.5, 261.6772) -> (-5.75, 261.6772)
  line L23 (-5.75, 261.6772) -> (-4.25, 263.7772)
  line L24 (-4.25, 263.7772) -> (-0.75, 263.7772)
  line L25 (-0.75, 263.7772) -> (0.75, 261.6772)
  line L26 (0.75, 261.6772) -> (2.5, 261.6772)
  line L27 (2.5, 261.6772) -> (4.25, 261.6772)
  line L28 (4.25, 261.6772) -> (5.75, 263.7772)
  line L29 (5.75, 263.7772) -> (9.25, 263.7772)
  line L30 (9.25, 263.7772) -> (10.75, 261.6772)
  line L31 (10.75, 261.6772) -> (12.5, 261.6772)
  line L32 (12.5, 261.6772) -> (14.25, 261.6772)
  line L33 (14.25, 261.6772) -> (15.75, 263.7772)
  line L34 (15.75, 263.7772) -> (19.25, 263.7772)
  line L35 (19.25, 263.7772) -> (20.75, 261.6772)
  line L36 (20.75, 261.6772) -> (22.5, 261.6772)
  line L37 (22.5, 261.6772) -> (24.25, 261.6772)
  line L38 (24.25, 261.6772) -> (25.75, 263.7772)
  line L39 (25.75, 263.7772) -> (29.25, 263.7772)
  line L40 (29.25, 263.7772) -> (30.75, 261.6772)
  line L41 (30.75, 261.6772) -> (32.5, 261.6772)
  line L42 (32.5, 261.6772) -> (34.25, 261.6772)
  line L43 (34.25, 261.6772) -> (35.75, 263.7772)
  line L44 (35.75, 263.7772) -> (39.25, 263.7772)
  line L45 (39.25, 263.7772) -> (40.75, 261.6772)
  line L46 (40.75, 261.6772) -> (42.5, 261.6772)
  line L47 (42.5, 261.6772) -> (44.25, 261.6772)
  line L48 (44.25, 261.6772) -> (45.75, 263.7772)
  line L49 (45.75, 263.7772) -> (49.25, 263.7772)
  line L50 (49.25, 263.7772) -> (50.75, 261.6772)
  line L51 (-50, 262.7272) -> (-49.25, 261.6772)
  line L52 (50.75, 261.6772) -> (54.25, 261.6772)
  line L53 (54.25, 261.6772) -> (55, 262.7272)
  line L54 (-49.9634, 262.7533) -> (-49.2268, 261.7222)
  line L55 (-49.2268, 261.7222) -> (-47.5, 261.7222)
  line L56 (-47.5, 261.7222) -> (-45.7732, 261.7222)
  line L57 (-45.7732, 261.7222) -> (-44.2732, 263.8222)
  line L58 (-44.2732, 263.8222) -> (-40.7268, 263.8222)
  line L59 (-40.7268, 263.8222) -> (-39.2268, 261.7222)
  line L60 (-39.2268, 261.7222) -> (-37.5, 261.7222)
  line L61 (-37.5, 261.7222) -> (-35.7732, 261.7222)
  line L62 (-35.7732, 261.7222) -> (-34.2732, 263.8222)
  line L63 (-34.2732, 263.8222) -> (-30.7268, 263.8222)
  line L64 (-30.7268, 263.8222) -> (-29.2268, 261.7222)
  line L65 (-29.2268, 261.7222) -> (-27.5, 261.7222)
  line L66 (-27.5, 261.7222) -> (-25.7732, 261.7222)
  line L67 (-25.7732, 261.7222) -> (-24.2732, 263.8222)
  line L68 (-24.2732, 263.8222) -> (-20.7268, 263.8222)
  line L69 (-20.7268, 263.8222) -> (-19.2268, 261.7222)
  line L70 (-19.2268, 261.7222) -> (-17.5, 261.7222)
  line L71 (-17.5, 261.7222) -> (-15.7732, 261.7222)
  line L72 (-15.7732, 261.7222) -> (-14.2732, 263.8222)
  line L73 (-14.2732, 263.8222) -> (-10.7268, 263.8222)
  line L74 (-10.7268, 263.8222) -> (-9.2268, 261.7222)
  line L75 (-9.2268, 261.7222) -> (-7.5, 261.7222)
  line L76 (-7.5, 261.7222) -> (-5.7732, 261.7222)
  line L77 (-5.7732, 261.7222) -> (-4.2732, 263.8222)
  line L78 (-4.2732, 263.8222) -> (-0.7268, 263.8222)
  line L79 (-0.7268, 263.8222) -> (0.7732, 261.7222)
  line L80 (0.7732, 261.7222) -> (2.5, 261.7222)
  line L81 (2.5, 261.7222) -> (4.2268, 261.7222)
  line L82 (4.2268, 261.7222) -> (5.7268, 263.8222)
  line L83 (5.7268, 263.8222) -> (9.2732, 263.8222)
  line L84 (9.2732, 263.8222) -> (10.7732, 261.7222)
  line L85 (10.7732, 261.7222) -> (12.5, 261.7222)
  line L86 (12.5, 261.7222) -> (14.2268, 261.7222)
  line L87 (14.2268, 261.7222) -> (15.7268, 263.8222)
  line L88 (15.7268, 263.8222) -> (19.2732, 263.8222)
  line L89 (19.2732, 263.8222) -> (20.7732, 261.7222)
  line L90 (20.7732, 261.7222) -> (22.5, 261.7222)
  line L91 (22.5, 261.7222) -> (24.2268, 261.7222)
  line L92 (24.2268, 261.7222) -> (25.7268, 263.8222)
  line L93 (25.7268, 263.8222) -> (29.2732, 263.8222)
  line L94 (29.2732, 263.8222) -> (30.7732, 261.7222)
  line L95 (30.7732, 261.7222) -> (32.5, 261.7222)
  line L96 (32.5, 261.7222) -> (34.2268, 261.7222)
  line L97 (34.2268, 261.7222) -> (35.7268, 263.8222)
  line L98 (35.7268, 263.8222) -> (39.2732, 263.8222)
  line L99 (39.2732, 263.8222) -> (40.7732, 261.7222)
  line L100 (40.7732, 261.7222) -> (42.5, 261.7222)
  line L101 (42.5, 261.7222) -> (44.2268, 261.7222)
  line L102 (44.2268, 261.7222) -> (45.7268, 263.8222)
  line L103 (45.7268, 263.8222) -> (49.2732, 263.8222)
  line L104 (49.2732, 263.8222) -> (50.7732, 261.7222)
  line L105 (50.7732, 261.7222) -> (54.2268, 261.7222)
  line L106 (54.2268, 261.7222) -> (54.9634, 262.7533)
  line L107 (-49.9634, 262.7533) -> (-50, 262.7272)
  line L108 (54.9634, 262.7533) -> (55, 262.7272)
  point P0 (550, 261.6772)
  point P1 (-49.25, 261.6772)
  point P2 (-47.5, 261.6772)
  point P3 (-45.75, 261.6772)
  point P4 (-39.25, 261.6772)
  point P5 (-37.5, 261.6772)
  point P6 (-35.75, 261.6772)
  point P7 (-42.5, 263.7772)
  point P8 (-44.25, 263.7772)
  point P9 (-40.75, 263.7772)
  point P10 (-50, 262.7272)
  point P11 (55, 262.7272)
  dimension "d225" = -0.045
  constraint coincident P1 L1.start
  constraint coincident P2 L1.end
  constraint coincident P3 L2.end
  constraint coincident P8 L3.end
  constraint coincident P9 L4.end
  constraint coincident P4 L5.end
  constraint coincident P10 L51.start
  constraint coincident P11 L53.end
  constraint perpendicular L51 L107
  constraint perpendicular L53 L108
extrude "Extrude1'''''''" add sketch "Sketch1 (8)" along normal blind 300 separate body makes body 104 in component "Крыша"
move_body "Move1''''''" bodies 104 to x (1, 0, 0) y (0, 1, 0) z (0, 0, 1) at (-294.4882, -57.2427, 0.75) in component "Крыша"
copy_body "CopyPasteBodies1''''" bodies 104 makes body 105 in component "Крыша"
move_body "Move2'''''''" bodies 105 to x (1, 0, 0) y (0, 1, 0) z (0, 0, 1) at (0, 0, -100) in component "Крыша"
copy_body "CopyPasteBodies2'''''" bodies 104 105 makes body 106 makes body 107 in component "Крыша"
move_body "Move3''''''" bodies 106 107 to x (1, 0, 0) y (0, 1, 0) z (0, 0, 1) at (0, 0, -200) in component "Крыша"
copy_body "CopyPasteBodies3'''''" bodies 104 105 makes body 108 makes body 109 in component "Крыша"
move_body "Move4'''''" bodies 108 109 to x (1, 0, 0) y (0, 1, 0) z (0, 0, 1) at (0, 0, -400) in component "Крыша"
sketch "Sketch1 (9)" plane through (5, 0, 0) normal (1, 0, 0) x (0, 0, -1) in component "Обшивка-Плиты"
  line L0 (0, 245.7192) -> (0, 20)
  line L1 (0, 20) -> (5, 20)
  line L2 (5, 20) -> (5, 245.7192)
  line L3 (5, 245.7192) -> (0, 245.7192)
  line L4 (0, 15) -> (125, 15)
  line L5 (125, 15) -> (125, 265)
  line L6 (125, 265) -> (0, 265)
  line L7 (0, 265) -> (0, 15)
  line L8 (500, 15) -> (250, 15)
  line L9 (250, 15) -> (250, 140)
  line L10 (250, 140) -> (500, 140)
  line L11 (500, 140) -> (500, 15)
  line L12 (500, 140) -> (250, 140)
  line L13 (250, 140) -> (250, 265)
  line L14 (250, 265) -> (500, 265)
  line L15 (500, 265) -> (500, 140)
  line L16 (125, 210.0714) -> (250, 210.0714)
  line L17 (250, 210.0714) -> (250, 265)
  line L18 (250, 265) -> (125, 265)
  line L19 (125, 265) -> (125, 210.0714)
  point P0 (0, 15)
  point P1 (500, 15)
  point P2 (125, 210.0714)
  dimension "d228" = 125
  dimension "d229" = 250
  dimension "d230" = 250
  dimension "d231" = 125
  dimension "d232" = 250
  dimension "d233" = 125
  dimension "d270" = 125
  constraint horizontal L4
  constraint vertical L5
  constraint horizontal L6
  constraint vertical L7
  constraint coincident P0 L4.start
  constraint horizontal L8
  constraint vertical L9
  constraint horizontal L10
  constraint vertical L11
  constraint coincident P1 L8.start
  constraint horizontal L12
  constraint vertical L13
  constraint horizontal L14
  constraint vertical L15
  constraint horizontal L16
  constraint vertical L17
  constraint horizontal L18
  constraint vertical L19
  constraint coincident L14 L13.end
  constraint coincident P2 L16.start
  measures "d228" distance of P0 L4.end
  measures "d229" distance of P0 L6.end
  measures "d230" distance of P1 L8.end
  measures "d231" distance of P1 L10.end
  measures "d232" distance of L10.end L9.end
  measures "d233" distance of L10.end L14.end
  measures "d270" distance of P2 L16.end
extrude "Extrude1''''''''" add sketch "Sketch1 (9)" along normal blind 1.12 separate body contours L0 L1 L2 L3 L7 | L1 L2 L3 L4 L5 L6 L7 L19 makes body 110 in component "Обшивка-Плиты"
extrude "Extrude4'''" add sketch "Sketch1 (9)" along normal blind 1.12 separate body contours L8 L9 L10 L11 L12 makes body 111 in component "Обшивка-Плиты"
extrude "Extrude5'''" add sketch "Sketch1 (9)" along normal blind 1.12 separate body contours L10 L12 L13 L14 L15 L17 makes body 112 in component "Обшивка-Плиты"
combine "Combine3'" operation cut target body 112 tool bodies 75 76 77 78 79 keep tools in component "Обшивка-Плиты"
combine "Combine4'" operation cut target body 110 tool bodies 72 73 71 keep tools in component "Обшивка-Плиты"